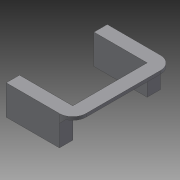
# Autodesk Inventor part: Fuse Box Support
Saved by Autodesk Inventor 2015 (Build 190159000, 159)
## iProperties
Created: 2017-12-29
Part Number: Fuse Box Support
Material: Generic
Document SubType Name: Modeling
Designer: Toby
Density: 1 g/cm^3
Appearance: Default
Author: Toby
Autodesk Inventor part; units mm, degrees
ref_plane "YZ Plane" through (0, 0, 0) normal (1, 0, 0) x (0, 1, 0)
ref_plane "XZ Plane" through (0, 0, 0) normal (0, 1, 0) x (-1, 0, 0)
ref_plane "XY Plane" through (0, 0, 0) normal (0, 0, 1) x (1, 0, 0)
sketch "Sketch1" plane through (0, 0, 0) normal (0, 0, 1) x (1, 0, 0)
  line L0 (-16.6287, 30.9385) -> (3.3713, 30.9385)
  line L1 (3.3713, 30.9385) -> (3.3713, 25.9385)
  line L2 (3.3713, 25.9385) -> (-16.6287, 25.9385)
  line L3 (-16.6287, 25.9385) -> (-16.6287, 30.9385)
  line L4 (-16.6287, -2.0615) -> (3.3713, -2.0615)
  line L5 (3.3713, -2.0615) -> (3.3713, -7.0615)
  line L6 (3.3713, -7.0615) -> (-16.6287, -7.0615)
  line L7 (-16.6287, -7.0615) -> (-16.6287, -2.0615)
  point P0 (0, 0)
  dimension "d0" = 20
  dimension "d1" = 5
  dimension "d2" = 5
  dimension "d3" = 20
  dimension "d4" = 38
  constraints: 16 end point, 4 parallel, 2 horizontal, 2 perpendicular, 1 point on line
  measures "d0" distance of L0.start L0.end
  measures "d1" distance of L2.end L0.start
  measures "d2" distance of L6.end L4.start
  measures "d3" distance of L4.start L4.end
  measures "d4" distance between parallel lines of L0 L6
extrude "Extrusion1" add sketch "Sketch1" along normal blind 10
sketch "Sketch2" plane through (0, 0, 10) normal (0, 0, 1) x (1, 0, 0)
  line L0 (-16.6287, 30.9385) -> (8.3713, 30.9385)
  line L1 (8.3713, 30.9385) -> (8.3713, -7.0615)
  line L2 (8.3713, -7.0615) -> (-16.6287, -7.0615)
  line L3 (-16.6287, -7.0615) -> (-16.6287, 30.9385)
  line L4 (-16.6287, -7.0615) -> (3.3713, -7.0615) projected
  point P0 (0, 0)
  dimension "d7" = 25
  constraints: 8 end point, 2 parallel, 1 collinear, 1 horizontal, 1 perpendicular
  measures "d7" distance between parallel lines of L3 L1
extrude "Extrusion2" add sketch "Sketch2" along normal blind 1.2
fillet "Fillet1" radius 5 2 edges at (8.3713, 30.9385, 10.6) (8.3713, -7.0615, 10.6)
chamfer "Chamfer1" distance 2 angle 45 2 edges at (3.3713, -4.5615, 10) (3.3713, 28.4385, 10)
sketch "Sketch3" plane through (0, 0, 10) normal (0, 0, -1) x (-1, 0, 0)
  line L0 (16.6287, -2.0615) -> (-3.3713, -2.0615)
  line L1 (-3.3713, -2.0615) -> (-3.3713, 25.9385)
  line L2 (-3.3713, 25.9385) -> (16.6287, 25.9385)
  line L3 (16.6287, 25.9385) -> (16.6287, -2.0615)
  point P0 (0, 0)
  constraints: 8 end point, 2 parallel, 1 horizontal, 1 perpendicular
extrude "Extrusion3" cut sketch "Sketch3" against normal blind 1.2
body "Solid1"
